Autodesk Inventor part; units mm, degrees
(part 2 of 2)
sketch "position草图" plane through (0, 8.5, 0) normal (0, 1, 0) x (1, 0, 0)
  line L0 (-87.5, 137.5) -> (-87.5, -137.5)
  line L1 (-87.5, 137.5) -> (-87.5, 91)
  line L2 (51.5, 137.5) -> (-87.5, 137.5)
  line L3 (51.5, -137.5) -> (51.5, 137.5)
  line L4 (-87.5, -137.5) -> (51.5, -137.5)
  circle A0 centre (-80.4289, -44.4289) radius 1.5 projected
  circle A1 centre (-40.4289, -130.4289) radius 1.5
  circle A2 centre (4.4289, -130.4289) radius 1.5
  circle A3 centre (4.4289, 130.4289) radius 1.5 projected
  circle A4 centre (-40.4289, 130.4289) radius 1.5 projected
  circle A5 centre (-80.4289, 44.4289) radius 1.5 projected
  circle A6 centre (-32.25, -132.9) radius 1.5
  circle A7 centre (-32.25, -102.7) radius 1.5
  circle A8 centre (-3.75, -132.9) radius 1.5
  circle A9 centre (-3.75, -102.7) radius 1.5
  line L5 (-85.025, -135.025) -> (-70.975, -135.025)
  line L6 (-70.975, -135.025) -> (-70.975, -120.975)
  line L7 (-70.975, -120.975) -> (-85.025, -120.975)
  line L8 (-85.025, -120.975) -> (-85.025, -135.025)
  line L9 (-85.025, -135.025) -> (-70.975, -120.975) construction
  line L10 (-70.975, -135.025) -> (-85.025, -120.975) construction
  line L11 (-85.025, -116.025) -> (-70.975, -116.025)
  line L12 (-70.975, -116.025) -> (-70.975, -101.975)
  line L13 (-70.975, -101.975) -> (-85.025, -101.975)
  line L14 (-85.025, -101.975) -> (-85.025, -116.025)
  line L15 (-85.025, -116.025) -> (-70.975, -101.975) construction
  line L16 (-70.975, -116.025) -> (-85.025, -101.975) construction
  line L17 (-85.025, -97.025) -> (-70.975, -97.025)
  line L18 (-70.975, -97.025) -> (-70.975, -82.975)
  line L19 (-70.975, -82.975) -> (-85.025, -82.975)
  line L20 (-85.025, -82.975) -> (-85.025, -97.025)
  line L21 (-85.025, -97.025) -> (-70.975, -82.975) construction
  line L22 (-70.975, -97.025) -> (-85.025, -82.975) construction
  line L23 (-85.025, -78.025) -> (-70.975, -78.025)
  line L24 (-70.975, -78.025) -> (-70.975, -63.975)
  line L25 (-70.975, -63.975) -> (-85.025, -63.975)
  line L26 (-85.025, -63.975) -> (-85.025, -78.025)
  line L27 (-85.025, -78.025) -> (-70.975, -63.975) construction
  line L28 (-70.975, -78.025) -> (-85.025, -63.975) construction
  line L29 (-51.0903, -62.4709) -> (-37.0403, -62.4709)
  line L30 (-37.0403, -62.4709) -> (-37.0403, -48.4209)
  line L31 (-37.0403, -48.4209) -> (-51.0903, -48.4209)
  line L32 (-51.0903, -48.4209) -> (-51.0903, -62.4709)
  line L33 (-51.0903, -62.4709) -> (-37.0403, -48.4209) construction
  line L34 (-37.0403, -62.4709) -> (-51.0903, -48.4209) construction
  line L35 (-47.0095, -39.3279) -> (-32.9595, -39.3279)
  line L36 (-32.9595, -39.3279) -> (-32.9595, -25.2779)
  line L37 (-32.9595, -25.2779) -> (-47.0095, -25.2779)
  line L38 (-47.0095, -25.2779) -> (-47.0095, -39.3279)
  line L39 (-47.0095, -39.3279) -> (-32.9595, -25.2779) construction
  line L40 (-32.9595, -39.3279) -> (-47.0095, -25.2779) construction
  line L41 (-33.5305, -20.0779) -> (-19.4805, -20.0779)
  line L42 (-19.4805, -20.0779) -> (-19.4805, -6.0279)
  line L43 (-19.4805, -6.0279) -> (-33.5305, -6.0279)
  line L44 (-33.5305, -6.0279) -> (-33.5305, -20.0779)
  line L45 (-33.5305, -20.0779) -> (-19.4805, -6.0279) construction
  line L46 (-19.4805, -20.0779) -> (-33.5305, -6.0279) construction
  line L47 (-31.3662, 6.6599) -> (-17.3162, 6.6599)
  line L48 (-17.3162, 6.6599) -> (-17.3162, 20.7099)
  line L49 (-17.3162, 20.7099) -> (-31.3662, 20.7099)
  line L50 (-31.3662, 20.7099) -> (-31.3662, 6.6599)
  line L51 (-31.3662, 6.6599) -> (-17.3162, 20.7099) construction
  line L52 (-17.3162, 6.6599) -> (-31.3662, 20.7099) construction
  line L53 (-45.7056, 27.1387) -> (-31.6556, 27.1387)
  line L54 (-31.6556, 27.1387) -> (-31.6556, 41.1887)
  line L55 (-31.6556, 41.1887) -> (-45.7056, 41.1887)
  line L56 (-45.7056, 41.1887) -> (-45.7056, 27.1387)
  line L57 (-45.7056, 27.1387) -> (-31.6556, 41.1887) construction
  line L58 (-31.6556, 27.1387) -> (-45.7056, 41.1887) construction
  line L59 (-54.2561, 50.6311) -> (-40.2061, 50.6311)
  line L60 (-40.2061, 50.6311) -> (-40.2061, 64.6811)
  line L61 (-40.2061, 64.6811) -> (-54.2561, 64.6811)
  line L62 (-54.2561, 64.6811) -> (-54.2561, 50.6311)
  line L63 (-54.2561, 50.6311) -> (-40.2061, 64.6811) construction
  line L64 (-40.2061, 50.6311) -> (-54.2561, 64.6811) construction
  line L65 (-56.435, 75.5359) -> (-42.385, 75.5359)
  line L66 (-42.385, 75.5359) -> (-42.385, 89.5859)
  line L67 (-42.385, 89.5859) -> (-56.435, 89.5859)
  line L68 (-56.435, 89.5859) -> (-56.435, 75.5359)
  line L69 (-56.435, 75.5359) -> (-42.385, 89.5859) construction
  line L70 (-42.385, 75.5359) -> (-56.435, 89.5859) construction
  line L71 (-78.8633, 64.7941) -> (-64.8133, 64.7941)
  line L72 (-64.8133, 64.7941) -> (-64.8133, 78.8441)
  line L73 (-64.8133, 78.8441) -> (-78.8633, 78.8441)
  line L74 (-78.8633, 78.8441) -> (-78.8633, 64.7941)
  line L75 (-78.8633, 64.7941) -> (-64.8133, 78.8441) construction
  line L76 (-64.8133, 64.7941) -> (-78.8633, 78.8441) construction
  line L77 (-76.6844, 39.8892) -> (-62.6344, 39.8892)
  line L78 (-62.6344, 39.8892) -> (-62.6344, 53.9392)
  line L79 (-62.6344, 53.9392) -> (-76.6844, 53.9392)
  line L80 (-76.6844, 53.9392) -> (-76.6844, 39.8892)
  line L81 (-76.6844, 39.8892) -> (-62.6344, 53.9392) construction
  line L82 (-62.6344, 39.8892) -> (-76.6844, 53.9392) construction
  line L83 (-68.1339, 16.3969) -> (-54.0839, 16.3969)
  line L84 (-54.0839, 16.3969) -> (-54.0839, 30.4469)
  line L85 (-54.0839, 30.4469) -> (-68.1339, 30.4469)
  line L86 (-68.1339, 30.4469) -> (-68.1339, 16.3969)
  line L87 (-68.1339, 16.3969) -> (-54.0839, 30.4469) construction
  line L88 (-54.0839, 16.3969) -> (-68.1339, 30.4469) construction
  line L89 (-53.7945, -4.0819) -> (-39.7445, -4.0819)
  line L90 (-39.7445, -4.0819) -> (-39.7445, 9.9681)
  line L91 (-39.7445, 9.9681) -> (-53.7945, 9.9681)
  line L92 (-53.7945, 9.9681) -> (-53.7945, -4.0819)
  line L93 (-53.7945, -4.0819) -> (-39.7445, 9.9681) construction
  line L94 (-39.7445, -4.0819) -> (-53.7945, 9.9681) construction
  line L95 (-78.6994, -6.2608) -> (-64.6494, -6.2608)
  line L96 (-64.6494, -6.2608) -> (-64.6494, 7.7892)
  line L97 (-64.6494, 7.7892) -> (-78.6994, 7.7892)
  line L98 (-78.6994, 7.7892) -> (-78.6994, -6.2608)
  line L99 (-78.6994, -6.2608) -> (-64.6494, 7.7892) construction
  line L100 (-64.6494, -6.2608) -> (-78.6994, 7.7892) construction
  line L101 (12.8421, -41.2372) -> (26.8921, -41.2372)
  line L102 (26.8921, -41.2372) -> (26.8921, -27.1872)
  line L103 (26.8921, -27.1872) -> (12.8421, -27.1872)
  line L104 (12.8421, -27.1872) -> (12.8421, -41.2372)
  line L105 (12.8421, -41.2372) -> (26.8921, -27.1872) construction
  line L106 (26.8921, -41.2372) -> (12.8421, -27.1872) construction
  line L107 (19.8671, -14.178) -> (33.9171, -14.178)
  line L108 (33.9171, -14.178) -> (33.9171, -0.128)
  line L109 (33.9171, -0.128) -> (19.8671, -0.128)
  line L110 (19.8671, -0.128) -> (19.8671, -14.178)
  line L111 (19.8671, -14.178) -> (33.9171, -0.128) construction
  line L112 (33.9171, -14.178) -> (19.8671, -0.128) construction
  line L113 (12.8421, 12.8811) -> (26.8921, 12.8811)
  line L114 (26.8921, 12.8811) -> (26.8921, 26.9311)
  line L115 (26.8921, 26.9311) -> (12.8421, 26.9311)
  line L116 (12.8421, 26.9311) -> (12.8421, 12.8811)
  line L117 (12.8421, 12.8811) -> (26.8921, 26.9311) construction
  line L118 (26.8921, 12.8811) -> (12.8421, 26.9311) construction
  line L119 (6.4757, 37.0569) -> (20.5257, 37.0569)
  line L120 (20.5257, 37.0569) -> (20.5257, 51.1069)
  line L121 (20.5257, 51.1069) -> (6.4757, 51.1069)
  line L122 (6.4757, 51.1069) -> (6.4757, 37.0569)
  line L123 (6.4757, 37.0569) -> (20.5257, 51.1069) construction
  line L124 (20.5257, 37.0569) -> (6.4757, 51.1069) construction
  line L125 (-39.9845, -32.3029) -> (-61.6957, -23.3099) projected
  line L126 (-68.7207, -30.3349) -> (-54.6707, -30.3349)
  line L127 (-54.6707, -30.3349) -> (-54.6707, -16.2849)
  line L128 (-54.6707, -16.2849) -> (-68.7207, -16.2849)
  line L129 (-68.7207, -16.2849) -> (-68.7207, -30.3349)
  line L130 (-68.7207, -30.3349) -> (-54.6707, -16.2849) construction
  line L131 (-54.6707, -30.3349) -> (-68.7207, -16.2849) construction
  line L132 (-28.75, -129.5) -> (-34.75, -129.5) projected
  line L133 (-28.75, -135.5) -> (-28.75, -129.5) projected
  line L134 (-34.75, -135.5) -> (-1.25, -135.5) projected
  line L135 (-34.75, -100.1) -> (-34.75, -135.5) projected
  line L136 (-28.75, -106.1) -> (-34.75, -106.1) projected
  line L137 (-28.75, -100.1) -> (-28.75, -106.1) projected
  line L138 (-34.75, -100.1) -> (-28.75, -100.1) projected
  line L139 (-34.75, -106.1) -> (-34.75, -100.1) projected
  line L140 (-7.25, -129.5) -> (-1.25, -129.5) projected
  line L141 (-7.25, -135.5) -> (-7.25, -129.5) projected
  line L142 (-1.25, -135.5) -> (-1.25, -100.1) projected
  line L143 (-7.25, -100.1) -> (-7.25, -106.1) projected
  line L144 (-7.25, -106.1) -> (-1.25, -106.1) projected
  line L145 (-1.25, -100.1) -> (-7.25, -100.1) projected
  line L146 (-1.25, -102.7) -> (-1.25, -100.1) projected
  line L147 (-1.25, -106.1) -> (-1.25, -100.1) projected
  line L148 (-1.25, -100.1) -> (-34.75, -100.1) projected
  point P0 (-78, -128)
  point P1 (-78, -109)
  point P2 (-78, -90)
  point P3 (-78, -71)
  point P4 (-44.0653, -55.4459)
  point P5 (-39.9845, -32.3029)
  point P6 (-26.5055, -13.0529)
  point P7 (-24.3412, 13.6849)
  point P8 (-38.6806, 34.1637)
  point P9 (-47.2311, 57.6561)
  point P10 (-49.41, 82.5609)
  point P11 (-71.8383, 71.8191)
  point P12 (-69.6594, 46.9142)
  point P13 (-61.1089, 23.4219)
  point P14 (-46.7695, 2.9431)
  point P15 (-71.6744, 0.7642)
  point P16 (19.8671, -34.2122)
  point P17 (26.8921, -7.153)
  point P18 (19.8671, 19.9061)
  point P19 (13.5007, 44.0819)
  dimension "d319" = 14.05
  dimension "d320" = 14.05
  dimension "d321" = 14.05
  dimension "d322" = 14.05
  dimension "d323" = 14.05
  dimension "d324" = 14.05
  dimension "d325" = 14.05
  dimension "d326" = 14.05
  dimension "d427" = 14.05
  dimension "d428" = 14.05
  dimension "d429" = 14.05
  dimension "d430" = 14.05
  dimension "d431" = 14.05
  dimension "d432" = 14.05
  dimension "d433" = 14.05
  dimension "d434" = 14.05
  dimension "d435" = 14.05
  dimension "d436" = 14.05
  dimension "d437" = 14.05
  dimension "d438" = 14.05
  dimension "d439" = 14.05
  dimension "d440" = 14.05
  dimension "d441" = 14.05
  dimension "d442" = 14.05
  dimension "d443" = 14.05
  dimension "d444" = 14.05
  dimension "d445" = 14.05
  dimension "d446" = 14.05
  dimension "d447" = 14.05
  dimension "d448" = 14.05
  dimension "d449" = 14.05
  dimension "d450" = 14.05
  dimension "d451" = 14.05
  dimension "d452" = 14.05
  dimension "d453" = 14.05
  dimension "d454" = 14.05
  dimension "d455" = 14.05
  dimension "d456" = 14.05
  dimension "d457" = 14.05
  dimension "d458" = 14.05
  dimension "d493" = 14.05
  dimension "d494" = 14.05
  constraints: 262 end point, 42 midpoint, 6 centre point
  measures "d319" distance of L7.end L6.end
  measures "d320" distance of L6.end L5.end
  measures "d321" distance of L13.end L12.end
  measures "d322" distance of L12.end L11.end
  measures "d323" distance of L19.end L18.end
  measures "d324" distance of L18.end L17.end
  measures "d325" distance of L25.end L24.end
  measures "d326" distance of L24.end L23.end
  measures "d427" distance of L31.end L30.end
  measures "d428" distance of L30.end L29.end
  measures "d429" distance of L37.end L36.end
  measures "d430" distance of L36.end L35.end
  measures "d431" distance of L43.end L42.end
  measures "d432" distance of L42.end L41.end
  measures "d433" distance of L49.end L48.end
  measures "d434" distance of L48.end L47.end
  measures "d435" distance of L55.end L54.end
  measures "d436" distance of L54.end L53.end
  measures "d437" distance of L61.end L60.end
  measures "d438" distance of L60.end L59.end
  measures "d439" distance of L67.end L66.end
  measures "d440" distance of L66.end L65.end
  measures "d441" distance of L73.end L72.end
  measures "d442" distance of L72.end L71.end
  measures "d443" distance of L79.end L78.end
  measures "d444" distance of L78.end L77.end
  measures "d445" distance of L85.end L84.end
  measures "d446" distance of L84.end L83.end
  measures "d447" distance of L91.end L90.end
  measures "d448" distance of L90.end L89.end
  measures "d449" distance of L97.end L96.end
  measures "d450" distance of L96.end L95.end
  measures "d451" distance of L103.end L102.end
  measures "d452" distance of L102.end L101.end
  measures "d453" distance of L109.end L108.end
  measures "d454" distance of L108.end L107.end
  measures "d455" distance of L115.end L114.end
  measures "d456" distance of L114.end L113.end
  measures "d457" distance of L121.end L120.end
  measures "d458" distance of L120.end L119.end
  measures "d493" distance of L128.end L127.end
  measures "d494" distance of L127.end L126.end
extrude "拉伸42" add sketch "position草图" against normal blind 1 separate body contours L2 L3 L4 L0 | A0 | A1 | A2 | A3 | A4 | A5 | A6 | A7 | A8 | A9 | L8 L7 L6 L5 | L14 L13 L12 L11 | L20 L19 L18 L17 | L26 L25 L24 L23 | L32 L31 L30 L29 | L38 L37 L36 L35 | L44 L43 L42 L41 | L50 L49 L48 L47 | L56 L55 L54 L53 | L62 L61 L60 L59 | L68 L67 L66 L65 | L74 L73 L72 L71 | L80 L79 L78 L77 | L86 L85 L84 L83 | L92 L91 L90 L89 | L98 L97 L96 L95 | L104 L103 L102 L101 | L110 L109 L108 L107 | L116 L115 L114 L113 | L122 L121 L120 L119 | L129 L128 L127 L126 | L133 L134 L135 L132 | L132 L135 L136 L137 L148 L143 L144 L142 L140 L141 L134 L133 | L135 L138 L137 L136 | L141 L140 L142 L134 | L145 L142 L144 L143
extrude "拉伸43" cut sketch "position草图" against normal through all contours L132 L135 L136 L137 L148 L143 L144 L142 L140 L141 L134 L133 bodies 7
extrude "拉伸44" cut sketch "position草图" against normal through all contours L8 L7 L6 L5 | L14 L13 L12 L11 | L20 L19 L18 L17 | L26 L25 L24 L23 | L32 L31 L30 L29 | L38 L37 L36 L35 | L44 L43 L42 L41 | L50 L49 L48 L47 | L56 L55 L54 L53 | L62 L61 L60 L59 | L68 L67 L66 L65 | L74 L73 L72 L71 | L80 L79 L78 L77 | L86 L85 L84 L83 | L92 L91 L90 L89 | L98 L97 L96 L95 | L104 L103 L102 L101 | L110 L109 L108 L107 | L116 L115 L114 L113 | L122 L121 L120 L119 | L129 L128 L127 L126 bodies 7
sketch "底板PCB定位孔草图" plane through (0, -2, 0) normal (0, -1, 0) x (1, 0, 0)
  circle A0 centre (-80.4289, -44.4289) radius 1.5 projected
  circle A1 centre (-80.4289, 44.4289) radius 1.5 projected
  circle A2 centre (-40.4289, 130.4289) radius 1.5 projected
  circle A3 centre (4.4289, 130.4289) radius 1.5 projected
  circle A4 centre (44.4289, 44.4289) radius 1.5 projected
  circle A5 centre (44.4289, -44.4289) radius 1.5 projected
  circle A6 centre (-40.4289, -130.4289) radius 1.5 projected
  circle A7 centre (-93.9645, -65.5355) radius 1.5 projected
  circle A8 centre (-93.9645, -87.4645) radius 1.5 projected
  circle A9 centre (-93.9645, -10.9645) radius 1.5 projected
  circle A10 centre (-93.9645, 10.9645) radius 1.5 projected
  circle A11 centre (-18.0001, -44.4289) radius 1.5 projected
  circle A12 centre (-18.0001, 44.4289) radius 1.5 projected
  circle A13 centre (4.4289, -130.4289) radius 1.5 projected
  point P0 (0, 0)
hole "底板PCB定位孔" at (-40.4289, -2, -130.4289) at (-80.4289, -2, -44.4289) at (-18.0001, -2, -44.4289) at (44.4289, -2, -44.4289) at (44.4289, -2, 44.4289) at (-18.0001, -2, 44.4289) at (-80.4289, -2, 44.4289) at (-40.4289, -2, 130.4289) at (4.4289, -2, 130.4289) at (-93.9645, -2, -87.4645) at (-93.9645, -2, -65.5355) at (-93.9645, -2, -10.9645) at (-93.9645, -2, 10.9645) at (4.4289, -2, -130.4289) direction (0, 1, 0) diameter 2.7 end through all counterbore diameter 5.6 counterbore depth 1 bodies 1 6 7
hole "OLED定位孔" at (-32.25, 8.5, 132.9) at (-32.25, 8.5, 102.7) at (-3.75, 8.5, 102.7) at (-3.75, 8.5, 132.9) direction (0, -1, 0) diameter 3.2 end through all bodies 7
sketch "PCB草图" plane through (0, 3.5, 0) normal (0, 1, 0) x (1, 0, 0)
  line L0 (-85.025, -120.975) -> (-85.025, -135.025) projected
  line L1 (-85.025, -135.025) -> (-70.975, -135.025) projected
  line L2 (-70.975, -120.975) -> (-85.025, -120.975) projected
  line L3 (-70.975, -135.025) -> (-70.975, -120.975) projected
  line L4 (-85.025, -135.025) -> (-70.975, -120.975) construction
  line L5 (-70.975, -135.025) -> (-85.025, -120.975) construction
  line L6 (-85.025, -116.025) -> (-70.975, -116.025) projected
  line L7 (-85.025, -101.975) -> (-85.025, -116.025) projected
  line L8 (-70.975, -101.975) -> (-85.025, -101.975) projected
  line L9 (-70.975, -116.025) -> (-70.975, -101.975) projected
  line L10 (-85.025, -116.025) -> (-70.975, -101.975) construction
  line L11 (-70.975, -116.025) -> (-85.025, -101.975) construction
  line L12 (-85.025, -82.975) -> (-85.025, -97.025) projected
  line L13 (-85.025, -97.025) -> (-70.975, -97.025) projected
  line L14 (-70.975, -97.025) -> (-70.975, -82.975) projected
  line L15 (-70.975, -82.975) -> (-85.025, -82.975) projected
  line L16 (-85.025, -97.025) -> (-70.975, -82.975) construction
  line L17 (-70.975, -97.025) -> (-85.025, -82.975) construction
  line L18 (-85.025, -78.025) -> (-70.975, -78.025) projected
  line L19 (-85.025, -63.975) -> (-85.025, -78.025) projected
  line L20 (-70.975, -63.975) -> (-85.025, -63.975) projected
  line L21 (-70.975, -78.025) -> (-70.975, -63.975) projected
  line L22 (-85.025, -78.025) -> (-70.975, -63.975) construction
  line L23 (-70.975, -78.025) -> (-85.025, -63.975) construction
  line L24 (-51.0903, -48.4209) -> (-51.0903, -62.4709) projected
  line L25 (-51.0903, -62.4709) -> (-37.0403, -62.4709) projected
  line L26 (-37.0403, -62.4709) -> (-37.0403, -48.4209) projected
  line L27 (-37.0403, -48.4209) -> (-51.0903, -48.4209) projected
  line L28 (-51.0903, -62.4709) -> (-37.0403, -48.4209) construction
  line L29 (-37.0403, -62.4709) -> (-51.0903, -48.4209) construction
  line L30 (-47.0095, -25.2779) -> (-47.0095, -39.3279) projected
  line L31 (-47.0095, -39.3279) -> (-32.9595, -39.3279) projected
  line L32 (-32.9595, -25.2779) -> (-47.0095, -25.2779) projected
  line L33 (-32.9595, -39.3279) -> (-32.9595, -25.2779) projected
  line L34 (-47.0095, -39.3279) -> (-32.9595, -25.2779) construction
  line L35 (-32.9595, -39.3279) -> (-47.0095, -25.2779) construction
  line L36 (-33.5305, -6.0279) -> (-33.5305, -20.0779) projected
  line L37 (-33.5305, -20.0779) -> (-19.4805, -20.0779) projected
  line L38 (-19.4805, -6.0279) -> (-33.5305, -6.0279) projected
  line L39 (-19.4805, -20.0779) -> (-19.4805, -6.0279) projected
  line L40 (-33.5305, -20.0779) -> (-19.4805, -6.0279) construction
  line L41 (-19.4805, -20.0779) -> (-33.5305, -6.0279) construction
  line L42 (-78.6994, 7.7892) -> (-78.6994, -6.2608) projected
  line L43 (-78.6994, -6.2608) -> (-64.6494, -6.2608) projected
  line L44 (-64.6494, 7.7892) -> (-78.6994, 7.7892) projected
  line L45 (-64.6494, -6.2608) -> (-64.6494, 7.7892) projected
  line L46 (-78.6994, -6.2608) -> (-64.6494, 7.7892) construction
  line L47 (-64.6494, -6.2608) -> (-78.6994, 7.7892) construction
  line L48 (-53.7945, 9.9681) -> (-53.7945, -4.0819) projected
  line L49 (-53.7945, -4.0819) -> (-39.7445, -4.0819) projected
  line L50 (-39.7445, 9.9681) -> (-53.7945, 9.9681) projected
  line L51 (-39.7445, -4.0819) -> (-39.7445, 9.9681) projected
  line L52 (-53.7945, -4.0819) -> (-39.7445, 9.9681) construction
  line L53 (-39.7445, -4.0819) -> (-53.7945, 9.9681) construction
  line L54 (-31.3662, 20.7099) -> (-31.3662, 6.6599) projected
  line L55 (-31.3662, 6.6599) -> (-17.3162, 6.6599) projected
  line L56 (-17.3162, 6.6599) -> (-17.3162, 20.7099) projected
  line L57 (-17.3162, 20.7099) -> (-31.3662, 20.7099) projected
  line L58 (-31.3662, 6.6599) -> (-17.3162, 20.7099) construction
  line L59 (-17.3162, 6.6599) -> (-31.3662, 20.7099) construction
  line L60 (-54.0839, 16.3969) -> (-54.0839, 30.4469) projected
  line L61 (-54.0839, 30.4469) -> (-68.1339, 30.4469) projected
  line L62 (-68.1339, 30.4469) -> (-68.1339, 16.3969) projected
  line L63 (-68.1339, 16.3969) -> (-54.0839, 16.3969) projected
  line L64 (-68.1339, 16.3969) -> (-54.0839, 30.4469) construction
  line L65 (-54.0839, 16.3969) -> (-68.1339, 30.4469) construction
  line L66 (-45.7056, 41.1887) -> (-45.7056, 27.1387) projected
  line L67 (-45.7056, 27.1387) -> (-31.6556, 27.1387) projected
  line L68 (-31.6556, 27.1387) -> (-31.6556, 41.1887) projected
  line L69 (-31.6556, 41.1887) -> (-45.7056, 41.1887) projected
  line L70 (-45.7056, 27.1387) -> (-31.6556, 41.1887) construction
  line L71 (-31.6556, 27.1387) -> (-45.7056, 41.1887) construction
  line L72 (-62.6344, 39.8892) -> (-62.6344, 53.9392) projected
  line L73 (-76.6844, 39.8892) -> (-62.6344, 39.8892) projected
  line L74 (-76.6844, 53.9392) -> (-76.6844, 39.8892) projected
  line L75 (-62.6344, 53.9392) -> (-76.6844, 53.9392) projected
  line L76 (-62.6344, 39.8892) -> (-76.6844, 53.9392) construction
  line L77 (-76.6844, 39.8892) -> (-62.6344, 53.9392) construction
  line L78 (-78.8633, 64.7941) -> (-64.8133, 64.7941) projected
  line L79 (-78.8633, 78.8441) -> (-78.8633, 64.7941) projected
  line L80 (-64.8133, 78.8441) -> (-78.8633, 78.8441) projected
  line L81 (-64.8133, 64.7941) -> (-64.8133, 78.8441) projected
  line L82 (-78.8633, 64.7941) -> (-64.8133, 78.8441) construction
  line L83 (-64.8133, 64.7941) -> (-78.8633, 78.8441) construction
  line L84 (-56.435, 89.5859) -> (-56.435, 75.5359) projected
  line L85 (-56.435, 75.5359) -> (-42.385, 75.5359) projected
  line L86 (-42.385, 75.5359) -> (-42.385, 89.5859) projected
  line L87 (-42.385, 89.5859) -> (-56.435, 89.5859) projected
  line L88 (-56.435, 75.5359) -> (-42.385, 89.5859) construction
  line L89 (-42.385, 75.5359) -> (-56.435, 89.5859) construction
  line L90 (12.8421, -27.1872) -> (12.8421, -41.2372) projected
  line L91 (12.8421, -41.2372) -> (26.8921, -41.2372) projected
  line L92 (26.8921, -41.2372) -> (26.8921, -27.1872) projected
  line L93 (26.8921, -27.1872) -> (12.8421, -27.1872) projected
  line L94 (12.8421, -41.2372) -> (26.8921, -27.1872) construction
  line L95 (26.8921, -41.2372) -> (12.8421, -27.1872) construction
  line L96 (19.8671, -0.128) -> (19.8671, -14.178) projected
  line L97 (19.8671, -14.178) -> (33.9171, -14.178) projected
  line L98 (33.9171, -14.178) -> (33.9171, -0.128) projected
  line L99 (33.9171, -0.128) -> (19.8671, -0.128) projected
  line L100 (19.8671, -14.178) -> (33.9171, -0.128) construction
  line L101 (33.9171, -14.178) -> (19.8671, -0.128) construction
  line L102 (12.8421, 12.8811) -> (26.8921, 12.8811) projected
  line L103 (12.8421, 26.9311) -> (12.8421, 12.8811) projected
  line L104 (26.8921, 26.9311) -> (12.8421, 26.9311) projected
  line L105 (26.8921, 12.8811) -> (26.8921, 26.9311) projected
  line L106 (12.8421, 12.8811) -> (26.8921, 26.9311) construction
  line L107 (26.8921, 12.8811) -> (12.8421, 26.9311) construction
  line L108 (6.4757, 37.0569) -> (20.5257, 37.0569) projected
  line L109 (6.4757, 51.1069) -> (6.4757, 37.0569) projected
  line L110 (20.5257, 51.1069) -> (6.4757, 51.1069) projected
  line L111 (20.5257, 37.0569) -> (20.5257, 51.1069) projected
  line L112 (6.4757, 37.0569) -> (20.5257, 51.1069) construction
  line L113 (20.5257, 37.0569) -> (6.4757, 51.1069) construction
  circle A0 centre (-40.4289, -130.4289) radius 1.5 projected
  circle A1 centre (4.4289, -130.4289) radius 1.5 projected
  circle A2 centre (44.4289, -44.4289) radius 1.35 projected
  circle A3 centre (-18.0001, -44.4289) radius 1.5 projected
  circle A4 centre (-80.4289, -44.4289) radius 1.5 projected
  circle A5 centre (-80.4289, 44.4289) radius 1.5 projected
  circle A6 centre (-18.0001, 44.4289) radius 1.5 projected
  circle A7 centre (44.4289, 44.4289) radius 1.5 projected
  circle A8 centre (-40.4289, 130.4289) radius 1.5 projected
  circle A9 centre (4.4289, 130.4289) radius 1.5 projected
  circle A10 centre (-93.9645, -10.9645) radius 1.5 projected
  circle A11 centre (-93.9645, 10.9645) radius 1.35 projected
  circle A12 centre (-93.9645, 65.5355) radius 1.35 projected
  circle A13 centre (-93.9645, 87.4645) radius 1.5 projected
  line L114 (-87.5, 91) -> (-97.5, 91)
  line L115 (-97.5, 91) -> (-97.5, 62)
  line L116 (-97.5, 62) -> (-87.5, 62)
  line L117 (-87.5, 62) -> (-87.5, 14.5)
  line L118 (-87.5, 14.5) -> (-97.5, 14.5)
  line L119 (-97.5, -14.5) -> (-97.5, 14.5)
  line L120 (-97.5, -14.5) -> (-87.5, -14.5)
  line L121 (-87.5, -14.5) -> (-87.5, -137.5)
  line L122 (-87.5, -137.5) -> (51.5, -137.5)
  line L123 (51.5, 137.5) -> (-87.5, 137.5)
  line L124 (-87.5, 137.5) -> (-87.5, 91)
  line L125 (-54.2561, 64.6811) -> (-54.2561, 50.6311) projected
  line L126 (-54.2561, 50.6311) -> (-40.2061, 50.6311) projected
  line L127 (-40.2061, 50.6311) -> (-40.2061, 64.6811) projected
  line L128 (-40.2061, 64.6811) -> (-54.2561, 64.6811) projected
  line L129 (-54.2561, 50.6311) -> (-40.2061, 64.6811) construction
  line L130 (-40.2061, 50.6311) -> (-54.2561, 64.6811) construction
  line L131 (51.5, 137.5) -> (31.5, 137.5)
  line L132 (51.5, 117.5) -> (51.5, 137.5)
  line L133 (51.5, 75.5) -> (51.5, 75.5359)
  line L134 (51.5, -117.5) -> (31.5, -117.5)
  line L135 (31.5, -117.5) -> (31.5, -97.5)
  line L136 (31.5, -97.5) -> (51.5, -97.5)
  line L137 (51.5, -137.5) -> (51.5, -117.5)
  line L138 (51.5, -97.5) -> (51.5, 137.5)
  line L139 (-68.7207, -16.2849) -> (-68.7207, -30.3349) projected
  line L140 (-68.7207, -30.3349) -> (-54.6707, -30.3349) projected
  line L141 (-54.6707, -30.3349) -> (-54.6707, -16.2849) projected
  line L142 (-54.6707, -16.2849) -> (-68.7207, -16.2849) projected
  line L143 (-68.7207, -30.3349) -> (-54.6707, -16.2849) construction
  line L144 (-54.6707, -30.3349) -> (-68.7207, -16.2849) construction
  line L145 (51.5, 137.5) -> (41.5, 137.5)
  line L146 (41.5, 137.5) -> (41.5, 117.5)
  line L147 (41.5, 117.5) -> (51.5, 117.5)
  line L148 (51.5, 117.5) -> (51.5, 137.5)
  line L149 (41.5, 117.5) -> (-10.5, 117.5)
  line L150 (-10.5, 117.5) -> (-10.5, 95.5)
  line L151 (-10.5, 95.5) -> (41.5, 95.5)
  line L152 (41.5, 95.5) -> (41.5, 117.5)
  circle A14 centre (-78, -128) radius 5
  circle A15 centre (-78, -109) radius 5
  circle A16 centre (-78, -90) radius 5
  circle A17 centre (-78, -71) radius 5
  circle A18 centre (-44.0653, -55.4459) radius 5
  circle A19 centre (-39.9845, -32.3029) radius 5
  circle A20 centre (-61.6957, -23.3099) radius 5
  circle A21 centre (-71.6744, 0.7642) radius 5
  circle A22 centre (-46.7695, 2.9431) radius 5
  circle A23 centre (-26.5055, -13.0529) radius 5
  circle A24 centre (-24.3412, 13.6849) radius 5
  circle A25 centre (-38.6806, 34.1637) radius 5
  circle A26 centre (-61.1089, 23.4219) radius 5
  circle A27 centre (-69.6594, 46.9142) radius 5
  circle A28 centre (-71.8383, 71.8191) radius 5
  circle A29 centre (-47.2311, 57.6561) radius 5
  circle A30 centre (-49.41, 82.5609) radius 5
  circle A31 centre (19.8671, -34.2122) radius 5
  circle A32 centre (26.8921, -7.153) radius 5
  circle A33 centre (19.8671, 19.9061) radius 5
  circle A34 centre (13.5007, 44.0819) radius 5
  point P0 (0, 0)
  dimension "d466" = 20
  dimension "d467" = 20
  dimension "d503" = 10
  dimension "d504" = 20
  dimension "d505" = 52
  dimension "d506" = 22
  dimension "d507" = 10
  dimension "d508" = 10
  dimension "d509" = 10
  dimension "d510" = 10
  dimension "d511" = 10
  dimension "d512" = 10
  dimension "d513" = 10
  dimension "d514" = 10
  dimension "d515" = 10
  dimension "d516" = 10
  dimension "d517" = 10
  dimension "d518" = 10
  dimension "d519" = 10
  dimension "d520" = 10
  dimension "d521" = 10
  dimension "d522" = 10
  dimension "d523" = 10
  dimension "d524" = 10
  dimension "d525" = 10
  dimension "d526" = 10
  dimension "d527" = 10
  constraints: 54 end point, 21 centre point, 2 point on line
  measures "d466" distance of L135.end L136.end
  measures "d467" distance of L134.end L135.end
  measures "d503" distance of L147.end L146.end
  measures "d504" distance of L146.end L145.end
  measures "d505" distance of L151.end L150.end
  measures "d506" distance of L150.end L149.end
  measures "d507" diameter of A14
  measures "d508" diameter of A15
  measures "d509" diameter of A16
  measures "d510" diameter of A17
  measures "d511" diameter of A18
  measures "d512" diameter of A19
  measures "d513" diameter of A20
  measures "d514" diameter of A21
  measures "d515" diameter of A22
  measures "d516" diameter of A23
  measures "d517" diameter of A24
  measures "d518" diameter of A25
  measures "d519" diameter of A26
  measures "d520" diameter of A27
  measures "d521" diameter of A28
  measures "d522" diameter of A29
  measures "d523" diameter of A30
  measures "d524" diameter of A31
  measures "d525" diameter of A32
  measures "d526" diameter of A33
  measures "d527" diameter of A34
thicken "加厚1" operation add thickness 1 both sides no extend neighbours no toward (1, 0, 0) bodies 3 faces at (-98, 6.6667, 8.2667)
thicken "加厚2" operation add thickness 1 both sides no extend neighbours no toward (1, 0, 0) bodies 3 faces at (-98, 6.6667, -11.6333)
thicken "加厚3" operation add thickness 1 both sides no extend neighbours no toward (1, 0, 0) bodies 3 faces at (-98, 6.6667, -68.2333)
thicken "加厚4" operation add thickness 1 both sides no extend neighbours no toward (1, 0, 0) bodies 3 faces at (-98, 6.6667, -88.1333)
thicken "加厚5" operation add thickness 1 both sides no extend neighbours no toward (1, 0, 0) bodies 2 faces at (-98, 2.6667, -5)
thicken "加厚6" operation add thickness 1 both sides no extend neighbours no toward (1, 0, 0) bodies 2 faces at (-98, 2.6667, -81.5)
sketch "PositionPlate_2D" plane through (0, 8.5, 0) normal (0, 1, 0) x (1, 0, 0)
  circle A0 centre (-3.75, -132.9) radius 1.6 projected
  circle A1 centre (-3.75, -102.7) radius 1.6 projected
  circle A2 centre (-32.25, -102.7) radius 1.6 projected
  circle A3 centre (-32.25, -132.9) radius 1.6 projected
  circle A4 centre (4.4289, 130.4289) radius 1.35 projected
  circle A5 centre (4.4289, -130.4289) radius 1.35 projected
  circle A6 centre (-40.4289, -130.4289) radius 1.35 projected
  circle A7 centre (-80.4289, -44.4289) radius 1.35 projected
  circle A8 centre (-18.0001, -44.4289) radius 1.35 projected
  circle A9 centre (44.4289, -44.4289) radius 1.35 projected
  circle A10 centre (44.4289, 44.4289) radius 1.35 projected
  circle A11 centre (-18.0001, 44.4289) radius 1.35 projected
  circle A12 centre (-80.4289, 44.4289) radius 1.35 projected
  circle A13 centre (-40.4289, 130.4289) radius 1.35 projected
  line L0 (-47.0095, -25.2779) -> (-32.9595, -25.2779) projected
  line L1 (-32.9595, -25.2779) -> (-32.9595, -39.3279) projected
  line L2 (-32.9595, -39.3279) -> (-47.0095, -39.3279) projected
  line L3 (-47.0095, -39.3279) -> (-47.0095, -25.2779) projected
  line L4 (-68.1339, 30.4469) -> (-54.0839, 30.4469) projected
  line L5 (-54.0839, 30.4469) -> (-54.0839, 16.3969) projected
  line L6 (-54.0839, 16.3969) -> (-68.1339, 16.3969) projected
  line L7 (-68.1339, 16.3969) -> (-68.1339, 30.4469) projected
  line L8 (-54.2561, 64.6811) -> (-40.2061, 64.6811) projected
  line L9 (-40.2061, 64.6811) -> (-40.2061, 50.6311) projected
  line L10 (-40.2061, 50.6311) -> (-54.2561, 50.6311) projected
  line L11 (-54.2561, 50.6311) -> (-54.2561, 64.6811) projected
  line L12 (19.8671, -0.128) -> (33.9171, -0.128) projected
  line L13 (33.9171, -0.128) -> (33.9171, -14.178) projected
  line L14 (33.9171, -14.178) -> (19.8671, -14.178) projected
  line L15 (19.8671, -14.178) -> (19.8671, -0.128) projected
  line L16 (-70.975, -101.975) -> (-70.975, -116.025) projected
  line L17 (-70.975, -116.025) -> (-85.025, -116.025) projected
  line L18 (-85.025, -116.025) -> (-85.025, -101.975) projected
  line L19 (-85.025, -101.975) -> (-70.975, -101.975) projected
  line L20 (-70.975, -82.975) -> (-70.975, -97.025) projected
  line L21 (-70.975, -97.025) -> (-85.025, -97.025) projected
  line L22 (-85.025, -97.025) -> (-85.025, -82.975) projected
  line L23 (-85.025, -82.975) -> (-70.975, -82.975) projected
  line L24 (12.8421, 26.9311) -> (26.8921, 26.9311) projected
  line L25 (26.8921, 26.9311) -> (26.8921, 12.8811) projected
  line L26 (26.8921, 12.8811) -> (12.8421, 12.8811) projected
  line L27 (12.8421, 12.8811) -> (12.8421, 26.9311) projected
  line L28 (-45.7056, 41.1887) -> (-31.6556, 41.1887) projected
  line L29 (-31.6556, 41.1887) -> (-31.6556, 27.1387) projected
  line L30 (-31.6556, 27.1387) -> (-45.7056, 27.1387) projected
  line L31 (-45.7056, 27.1387) -> (-45.7056, 41.1887) projected
  line L32 (-76.6844, 53.9392) -> (-62.6344, 53.9392) projected
  line L33 (-62.6344, 53.9392) -> (-62.6344, 39.8892) projected
  line L34 (-62.6344, 39.8892) -> (-76.6844, 39.8892) projected
  line L35 (-76.6844, 39.8892) -> (-76.6844, 53.9392) projected
  line L36 (-33.5305, -6.0279) -> (-19.4805, -6.0279) projected
  line L37 (-19.4805, -6.0279) -> (-19.4805, -20.0779) projected
  line L38 (-19.4805, -20.0779) -> (-33.5305, -20.0779) projected
  line L39 (-33.5305, -20.0779) -> (-33.5305, -6.0279) projected
  line L40 (-51.0903, -48.4209) -> (-37.0403, -48.4209) projected
  line L41 (-37.0403, -48.4209) -> (-37.0403, -62.4709) projected
  line L42 (-37.0403, -62.4709) -> (-51.0903, -62.4709) projected
  line L43 (-51.0903, -62.4709) -> (-51.0903, -48.4209) projected
  line L44 (-78.6994, 7.7892) -> (-64.6494, 7.7892) projected
  line L45 (-64.6494, 7.7892) -> (-64.6494, -6.2608) projected
  line L46 (-64.6494, -6.2608) -> (-78.6994, -6.2608) projected
  line L47 (-78.6994, -6.2608) -> (-78.6994, 7.7892) projected
  line L48 (-56.435, 89.5859) -> (-42.385, 89.5859) projected
  line L49 (-42.385, 89.5859) -> (-42.385, 75.5359) projected
  line L50 (-42.385, 75.5359) -> (-56.435, 75.5359) projected
  line L51 (-56.435, 75.5359) -> (-56.435, 89.5859) projected
  line L52 (12.8421, -27.1872) -> (26.8921, -27.1872) projected
  line L53 (26.8921, -27.1872) -> (26.8921, -41.2372) projected
  line L54 (26.8921, -41.2372) -> (12.8421, -41.2372) projected
  line L55 (12.8421, -41.2372) -> (12.8421, -27.1872) projected
  line L56 (-85.025, -135.025) -> (-85.025, -120.975) projected
  line L57 (-85.025, -120.975) -> (-70.975, -120.975) projected
  line L58 (-70.975, -120.975) -> (-70.975, -135.025) projected
  line L59 (-70.975, -135.025) -> (-85.025, -135.025) projected
  line L60 (-70.975, -63.975) -> (-70.975, -78.025) projected
  line L61 (-70.975, -78.025) -> (-85.025, -78.025) projected
  line L62 (-85.025, -78.025) -> (-85.025, -63.975) projected
  line L63 (-85.025, -63.975) -> (-70.975, -63.975) projected
  line L64 (6.4757, 51.1069) -> (20.5257, 51.1069) projected
  line L65 (20.5257, 51.1069) -> (20.5257, 37.0569) projected
  line L66 (20.5257, 37.0569) -> (6.4757, 37.0569) projected
  line L67 (6.4757, 37.0569) -> (6.4757, 51.1069) projected
  line L68 (-31.3662, 20.7099) -> (-17.3162, 20.7099) projected
  line L69 (-17.3162, 20.7099) -> (-17.3162, 6.6599) projected
  line L70 (-17.3162, 6.6599) -> (-31.3662, 6.6599) projected
  line L71 (-31.3662, 6.6599) -> (-31.3662, 20.7099) projected
  line L72 (-78.8633, 78.8441) -> (-64.8133, 78.8441) projected
  line L73 (-64.8133, 78.8441) -> (-64.8133, 64.7941) projected
  line L74 (-64.8133, 64.7941) -> (-78.8633, 64.7941) projected
  line L75 (-78.8633, 64.7941) -> (-78.8633, 78.8441) projected
  line L76 (-53.7945, 9.9681) -> (-39.7445, 9.9681) projected
  line L77 (-39.7445, 9.9681) -> (-39.7445, -4.0819) projected
  line L78 (-39.7445, -4.0819) -> (-53.7945, -4.0819) projected
  line L79 (-53.7945, -4.0819) -> (-53.7945, 9.9681) projected
  line L80 (-68.7207, -16.2849) -> (-54.6707, -16.2849) projected
  line L81 (-54.6707, -16.2849) -> (-54.6707, -30.3349) projected
  line L82 (-54.6707, -30.3349) -> (-68.7207, -30.3349) projected
  line L83 (-68.7207, -30.3349) -> (-68.7207, -16.2849) projected
  line L84 (-34.75, -106.1) -> (-28.75, -106.1) projected
  line L85 (-28.75, -106.1) -> (-28.75, -100.1) projected
  line L86 (-28.75, -100.1) -> (-7.25, -100.1) projected
  line L87 (-7.25, -100.1) -> (-7.25, -106.1) projected
  line L88 (-7.25, -106.1) -> (-1.25, -106.1) projected
  line L89 (-1.25, -106.1) -> (-1.25, -129.5) projected
  line L90 (-1.25, -129.5) -> (-7.25, -129.5) projected
  line L91 (-7.25, -129.5) -> (-7.25, -135.5) projected
  line L92 (-7.25, -135.5) -> (-28.75, -135.5) projected
  line L93 (-28.75, -135.5) -> (-28.75, -129.5) projected
  line L94 (-28.75, -129.5) -> (-34.75, -129.5) projected
  line L95 (-34.75, -129.5) -> (-34.75, -106.1) projected
  line L96 (-87.5, 137.5) -> (-87.5, -137.5) projected
  line L97 (-87.5, -137.5) -> (51.5, -137.5) projected
  line L98 (51.5, -137.5) -> (51.5, 137.5) projected
  line L99 (51.5, 137.5) -> (-87.5, 137.5) projected
  point P0 (0, 0)
